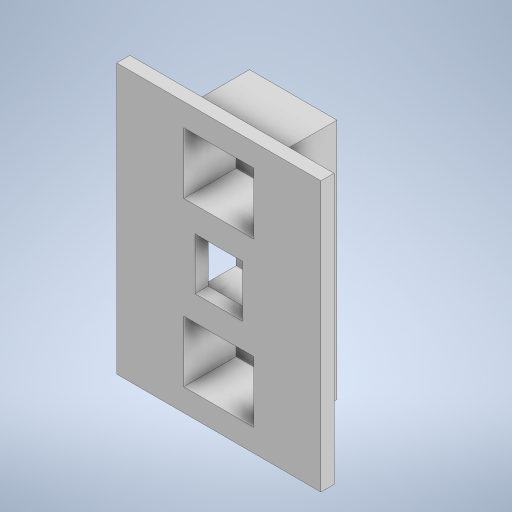
# Autodesk Inventor part: newairtempguytop
Saved by Autodesk Inventor 2023 (Build 270158000, 158)
## iProperties
Created: 2023-02-08
Part Number: newairtempguytop
Material: Generic
Document SubType Name: Modeling
Designer: efarq
Density: 1 g/cm^3
Appearance: Default
Author: efarq
Autodesk Inventor part; units mm, degrees
ref_plane "Work Plane3" through (0, 0, 3.5) normal (0, 0, 1) x (1, 0, 0)
sketch "Sketch2" plane through (0, 0, 3.5) normal (0, 0, 1) x (1, 0, 0)
  line L0 (-11.6713, -15.4051) -> (11.6713, -15.4051)
  line L1 (11.6713, -15.4051) -> (11.6713, 15.4051)
  line L2 (11.6713, 15.4051) -> (-11.6713, 15.4051)
  line L3 (-11.6713, 15.4051) -> (-11.6713, -15.4051)
  line L4 (-11.6713, -15.4051) -> (11.6713, 15.4051) construction
  line L5 (11.6713, -15.4051) -> (-11.6713, 15.4051) construction
  point P0 (0, 0)
  dimension "d4" = 30.8102
  dimension "d5" = 23.3426
  constraints: 12 end point, 2 midpoint, 2 parallel, 1 horizontal, 1 perpendicular
  measures "d4" distance of L0.end L1.end
  measures "d5" distance of L1.end L2.end
extrude "Extrusion2" add sketch "Sketch2" along normal blind 1.5
ref_plane "Work Plane2" through (0, 0, 0) normal (0, 0, -1) x (-1, 0, 0)
sketch "Sketch3" plane through (0, 0, 0) normal (0, 0, -1) x (-1, 0, 0)
  line L0 (-2.7149, 2.9592) -> (2.7149, 2.9592)
  line L1 (2.7149, 2.9592) -> (2.7149, -2.9592)
  line L2 (2.7149, -2.9592) -> (-2.7149, -2.9592)
  line L3 (-2.7149, -2.9592) -> (-2.7149, 2.9592)
  line L4 (-2.7149, 2.9592) -> (2.7149, -2.9592) construction
  line L5 (2.7149, 2.9592) -> (-2.7149, -2.9592) construction
  point P0 (0, 0)
  constraints: 12 end point, 2 midpoint, 2 parallel, 1 horizontal, 1 perpendicular
extrude "Extrusion3" cut sketch "Sketch3" against normal blind 6
ref_plane "Work Plane1" through (0, 0, 0) normal (0, 0, -1) x (-1, 0, 0)
sketch "Sketch4" plane through (0, 0, 0) normal (0, 0, -1) x (-1, 0, 0)
  line L0 (8.89, -12.7) -> (-8.89, -12.7) projected
  line L1 (3.6472, 12.7) -> (-3.3528, 12.7)
  line L2 (-3.3528, 12.7) -> (-3.3528, 7.7)
  line L3 (-3.3528, 7.7) -> (3.6472, 7.7)
  line L4 (3.6472, 7.7) -> (3.6472, 12.7)
  line L5 (3.6472, 12.7) -> (-3.3528, 7.7) construction
  line L6 (-3.3528, 12.7) -> (3.6472, 7.7) construction
  line L7 (-8.89, -12.7) -> (-8.89, 12.7) projected
  line L8 (3.6472, -7.7) -> (-3.3528, -7.7)
  line L9 (-3.3528, -7.7) -> (-3.3528, -12.7)
  line L10 (-3.3528, -12.7) -> (3.6472, -12.7)
  line L11 (3.6472, -12.7) -> (3.6472, -7.7)
  line L12 (3.6472, -7.7) -> (-3.3528, -12.7) construction
  line L13 (-3.3528, -7.7) -> (3.6472, -12.7) construction
  line L14 (-8.89, 12.7) -> (8.89, 12.7) projected
  point P0 (0, 0)
  point P1 (0.1472, 10.2)
  point P2 (0.1472, -10.2)
  point P3 (-3.3528, -10.2)
  dimension "d10" = 7
  dimension "d11" = 5
  dimension "d12" = 5.5372
  dimension "d13" = 7
  dimension "d14" = 5
  dimension "d15" = 5.5372
  dimension "d16" = 0
  dimension "d17" = 0
  constraints: 24 end point, 5 midpoint, 4 parallel, 2 horizontal, 2 perpendicular
  measures "d10" distance of L1.start L1.end
  measures "d11" distance of L1.end L2.end
  measures "d12" distance between parallel lines of L2 L7
  measures "d13" distance of L8.start L8.end
  measures "d14" distance of L8.end L9.end
  measures "d15" distance from line of L7 point (-3.353, -10.2)
  measures "d16" distance between parallel lines of L0 L10
  measures "d17" distance between parallel lines of L14 L1
extrude "Extrusion4" cut sketch "Sketch4" against normal blind 3.5
sketch "Sketch5" plane through (0, 0, 3.5) normal (0, 0, -1) x (-1, 0, 0)
  line L0 (11.6713, -15.4051) -> (-11.6713, -15.4051) projected
  line L1 (-4.0005, -12.827) -> (3.9995, -12.827)
  line L2 (3.9995, -12.827) -> (3.9995, -5.827)
  line L3 (3.9995, -5.827) -> (-4.0005, -5.827)
  line L4 (-4.0005, -5.827) -> (-4.0005, -12.827)
  line L5 (-11.6713, -15.4051) -> (-11.6713, 15.4051) projected
  line L6 (2.7149, -2.9592) -> (-2.7149, -2.9592) projected
  line L7 (9.017, -12.827) -> (-9.017, -12.827)
  line L8 (-9.017, -12.827) -> (-9.017, 12.827)
  line L9 (-9.017, 12.827) -> (9.017, 12.827)
  line L10 (9.017, 12.827) -> (9.017, -12.827)
  line L11 (9.017, -12.827) -> (-9.017, 12.827) construction
  line L12 (-9.017, -12.827) -> (9.017, 12.827) construction
  line L13 (3.9995, 5.827) -> (-4.0005, 5.827)
  line L14 (-4.0005, 5.827) -> (-4.0005, 12.827)
  line L15 (-4.0005, 12.827) -> (3.9995, 12.827)
  line L16 (3.9995, 12.827) -> (3.9995, 5.827)
  line L17 (3.9995, 5.827) -> (-4.0005, 12.827) construction
  line L18 (-4.0005, 5.827) -> (3.9995, 12.827) construction
  line L19 (11.6713, 15.4051) -> (11.6713, -15.4051) projected
  point P0 (0, 0)
  point P1 (-0.0005, 9.327)
  point P2 (3.9995, 12.827)
  dimension "d20" = 8
  dimension "d21" = 7
  dimension "d22" = 7.6708
  dimension "d25" = 18.034
  dimension "d26" = 25.654
  dimension "d27" = 0
  dimension "d28" = 7
  dimension "d29" = 8
  dimension "d31" = 7.6718
  constraints: 32 end point, 6 parallel, 4 midpoint, 3 horizontal, 3 perpendicular, 1 point on line
  measures "d20" distance of L3.end L2.end
  measures "d21" distance of L1.end L2.end
  measures "d22" distance between parallel lines of L5 L4
  measures "d25" distance of L8.end L9.end
  measures "d26" distance of L7.end L8.end
  measures "d27" distance between parallel lines of L7 L1
  measures "d28" distance of L13.end L14.end
  measures "d29" distance of L13.start L13.end
  measures "d31" distance between parallel lines of L19 L16
extrude "Extrusion5" add sketch "Sketch5" along normal blind 4.5 contours L4 L3 L2 L1 | L9 L16 L13 L14
sketch "Sketch6" plane through (0, 0, -1) normal (0, 0, -1) x (-1, 0, 0)
  line L0 (4.9995, 13.827) -> (-5.0005, 13.827)
  line L1 (-5.0005, 13.827) -> (-5.0005, 4.827)
  line L2 (-5.0005, 4.827) -> (4.9995, 4.827)
  line L3 (4.9995, 4.827) -> (4.9995, 13.827)
  line L4 (4.9995, -4.827) -> (-5.0005, -4.827)
  line L5 (-5.0005, -4.827) -> (-5.0005, -13.827)
  line L6 (-5.0005, -13.827) -> (4.9995, -13.827)
  line L7 (4.9995, -13.827) -> (4.9995, -4.827)
  line L8 (-4.0005, 5.827) -> (3.9995, 5.827) projected
  line L9 (3.9995, 12.827) -> (-4.0005, 12.827) projected
  line L10 (3.9995, 5.827) -> (3.9995, 12.827) projected
  line L11 (-4.0005, 12.827) -> (-4.0005, 5.827) projected
  line L12 (-4.0005, -12.827) -> (3.9995, -12.827) projected
  line L13 (3.9995, -5.827) -> (-4.0005, -5.827) projected
  point P0 (0, 0)
  dimension "d35" = 1
  dimension "d36" = 1
  dimension "d37" = 1
  dimension "d38" = 1
  dimension "d39" = 1
  dimension "d40" = 1
  constraints: 16 end point, 4 parallel, 2 horizontal, 2 perpendicular, 2 point on line
  measures "d35" distance between parallel lines of L2 L8
  measures "d36" distance between parallel lines of L9 L0
  measures "d37" distance between parallel lines of L10 L3
  measures "d38" distance between parallel lines of L11 L1
  measures "d39" distance between parallel lines of L6 L12
  measures "d40" distance between parallel lines of L4 L13
extrude "Extrusion6" add sketch "Sketch6" along normal blind 1 and the other way blind 4.5 contours L3 L2 L1 L0 | L7 L6 L5 L4 | L11 L9 L10 L8
extrude "Extrusion7" cut sketch "Sketch5" along normal blind 4.5 and the other way blind 1.5 contours L4 L3 L2 L1 | L9 L16 L13 L14
sketch "Sketch8" plane through (0, 0, -2) normal (0, 0, -1) x (-1, 0, 0)
  line L0 (4.9995, 13.827) -> (4.9995, 4.827) projected
  line L1 (-5.0005, -13.827) -> (4.9995, -13.827) projected
  line L2 (4.9995, 13.827) -> (-5.0005, 13.827)
  line L3 (-5.0005, 13.827) -> (-5.0005, -13.827)
  line L4 (-5.0005, -13.827) -> (4.9995, -13.827)
  line L5 (4.9995, -13.827) -> (4.9995, 13.827)
  point P0 (0, 0)
  constraints: 8 end point, 2 parallel, 1 horizontal, 1 perpendicular
extrude "Extrusion8" add sketch "Sketch8" along normal blind 1.5
body "Solid1"
